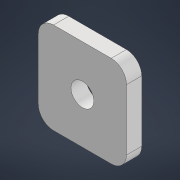
# Autodesk Inventor part: mount_linear_stepper_washer_b
Saved by Autodesk Inventor 2021 (Build 250183000, 183)
## iProperties
Created: 2020-12-29
Part Number: mount_linear_stepper_washer_b
Material: Generic
Document SubType Name: Modeling
Designer: Tomasz
Density: 1 g/cm^3
Appearance: Default
Author: Tomasz
Autodesk Inventor part; units mm, degrees
ref_plane "YZ Plane" through (0, 0, 0) normal (1, 0, 0) x (0, 1, 0)
ref_plane "XZ Plane" through (0, 0, 0) normal (0, 1, 0) x (-1, 0, 0)
ref_plane "XY Plane" through (0, 0, 0) normal (0, 0, 1) x (1, 0, 0)
sketch "washer_sketch" plane through (0, 0, 0) normal (0, 0, 1) x (1, 0, 0)
  line L0 (-5.3709, -5.3107) -> (-5.3709, 4.5904) construction
  line L1 (0.3709, -5.3107) -> (-5.3709, -5.3107) construction
  arc A0 (0.3709, -5.3107) -> (5.3709, -0.3107) centre (0.3709, -0.3107) ccw construction
  arc A1 (5.3709, -0.3107) -> (-3.0036, 4.5904) centre (-0.2505, -0.3107) ccw construction
  line L2 (-5.3709, 4.5904) -> (-3.0036, 4.5904) construction
  circle A2 centre (0.4177, -0.0104) radius 3.55 construction
  circle A3 centre (0.4177, -0.0104) radius 3.55 construction
  circle A4 centre (0.4177, -0.0104) radius 1.5 projected
  line L3 (4.2064, 5.9896) -> (-3.3709, 5.9896)
  line L4 (-5.3709, 3.9896) -> (-5.3709, -4.0104)
  line L5 (-3.3709, -6.0104) -> (4.2064, -6.0104)
  line L6 (6.2064, -4.0104) -> (6.2064, 3.9896)
  arc A5 (6.2064, 3.9896) -> (4.2064, 5.9896) centre (4.2064, 3.9896) ccw
  arc A6 (4.2064, -6.0104) -> (6.2064, -4.0104) centre (4.2064, -4.0104) ccw
  arc A7 (-5.3709, -4.0104) -> (-3.3709, -6.0104) centre (-3.3709, -4.0104) ccw
  arc A8 (-3.3709, 5.9896) -> (-5.3709, 3.9896) centre (-3.3709, 3.9896) ccw
  point P0 (0, 0)
  point P1 (6.2064, 5.9896)
  point P2 (-5.3709, 5.9896)
  point P3 (6.2064, -6.0104)
  dimension "d0" = 12
  dimension "d1" = 11.5773
  dimension "d2" = 5.7886
  dimension "d3" = 6
  dimension "d4" = 2
  constraints: 8 end point, 8 point on circle, 8 tangent, 6 point on line, 4 centre point, 3 equal radius, 2 parallel, 1 horizontal, 1 perpendicular, 1 vertical alignment
  measures "d0" distance of point (6.206, -6.01) point (6.206, 5.99)
  measures "d1" distance of point (6.206, 5.99) point (-5.371, 5.99)
  measures "d2" distance from line of L0 A2.centre
  measures "d3" distance from line of A2.centre L3
  measures "d4" radius of A5
extrude "washer" add sketch "washer_sketch" along normal blind 2
equation "\"d1\" = 2 * d2"
equation "\"d3\" = 0.5 * d0"
body "Solid1"
